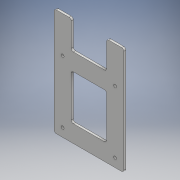
# Autodesk Inventor part: targetpart
Saved by Autodesk Inventor 2018 (Build 220112000, 112)
## iProperties
Created: 2018-05-08
Part Number: targetpart
Material: Generic
Document SubType Name: Modeling
Designer: alexs
Density: 1 g/cm^3
Appearance: Default
Author: alexs
Autodesk Inventor part; units mm, degrees
ref_plane "YZ Plane" through (0, 0, 0) normal (1, 0, 0) x (0, 1, 0)
ref_plane "XZ Plane" through (0, 0, 0) normal (0, 1, 0) x (-1, 0, 0)
ref_plane "XY Plane" through (0, 0, 0) normal (0, 0, 1) x (1, 0, 0)
sketch "Sketch1" plane through (0, 0, 0) normal (0, 1, 0) x (-1, 0, 0)
  line L0 (65, 0) -> (65, -100)
  line L1 (65, -100) -> (0, -100)
  line L2 (0, -100) -> (0, 0)
  line L3 (8, -34) -> (57, -34) construction
  line L4 (57, -34) -> (57, -92) construction
  line L5 (57, -92) -> (8, -92) construction
  line L6 (8, -92) -> (8, -34) construction
  circle A0 centre (57, -34) radius 1.35
  circle A1 centre (57, -92) radius 1.35
  circle A2 centre (8, -34) radius 1.35
  circle A3 centre (8, -92) radius 1.35
  line L7 (49, -42) -> (16, -42)
  line L8 (16, -42) -> (16, -84)
  line L9 (16, -84) -> (49, -84)
  line L10 (49, -84) -> (49, -42)
  line L11 (49, 0) -> (16, 0) construction
  line L12 (16, 0) -> (16, -26)
  line L13 (16, -26) -> (49, -26)
  line L14 (49, -26) -> (49, 0)
  line L15 (0, 0) -> (16, 0)
  line L16 (49, 0) -> (65, 0)
  point P0 (32.5, -34)
  dimension "d0" = 49
  dimension "d1" = 58
  dimension "d2" = 2.7
  dimension "d3" = 100
  dimension "d4" = 65
  dimension "d5" = 8
  dimension "d7" = 8
  dimension "d8" = 8
  dimension "d9" = 8
  dimension "d10" = 8
  dimension "d11" = 8
  dimension "d15" = 8
  constraints: 34 end point, 9 parallel, 5 horizontal, 5 perpendicular, 4 centre point, 4 coincident, 3 equal radius, 2 collinear, 1 midpoint
  measures "d0" distance of L4.end L5.end
  measures "d1" distance of L5.end L3.start
  measures "d2" diameter of A0
  measures "d3" distance of L0.start L0.end
  measures "d4" distance of L0.end L1.end
  measures "d5" distance between parallel lines of L2 L6
  measures "d7" distance from line of L1 A1.centre
  measures "d8" distance between parallel lines of L4 L10
  measures "d9" distance between parallel lines of L3 L7
  measures "d10" distance between parallel lines of L6 L8
  measures "d11" distance between parallel lines of L9 L5
  measures "d15" distance between parallel lines of L3 L13
extrude "Extrusion1" add sketch "Sketch1" along normal blind 2
fillet "Fillet1" radius 2 12 edges at (-49, 1, -84) (-49, 1, -42) (-16, 1, -42) (-16, 1, -84) (-65, 1, -100) (0, 1, -100) (0, 1, 0) (-65, 1, 0) (-49, 1, 0) (-49, 1, -26) (-16, 1, -26) (-16, 1, 0)
equation "\"d5\" = -0.5 * d0 + 0.5 * d4"
equation "\"d7\" = d5"
equation "\"d8\" = d5"
equation "\"d9\" = d5"
equation "\"d10\" = d5"
equation "\"d11\" = d5"
equation "\"d15\" = d5"
body "Solid1"
